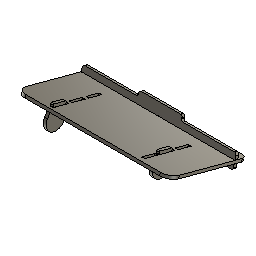
Stand3 (Autodesk Fusion 360 design; units mm, degrees)
Autodesk Fusion 360 part; units mm, degrees
note: some values were not read from the file. Set by a fixed rule: which sketch regions a step uses.
sketch "スケッチ1" plane through (0, 0, 0) normal (0, 0, 1) x (1, 0, 0) in component "base1"
  line L0 (0, 0) -> (160, 0)
  line L1 (160, 0) -> (160, 70)
  line L2 (160, 70) -> (0, 70) construction
  line L3 (0, 70) -> (0, 0)
  line L4 (0, 70) -> (160, 70) construction
  line L5 (160, 70) -> (160, 83)
  line L6 (160, 83) -> (0, 83)
  line L7 (0, 83) -> (0, 70)
  line L8 (80, 70) -> (0, 70)
  line L9 (0, 70) -> (0, 73)
  line L10 (0, 73) -> (80, 73)
  line L11 (80, 73) -> (80, 70)
  line L12 (32, 24) -> (35, 24)
  line L13 (35, 24) -> (35, 38)
  line L14 (35, 38) -> (32, 38)
  line L15 (32, 38) -> (32, 24)
  line L16 (32, 6) -> (35, 6)
  line L17 (35, 6) -> (35, 20)
  line L18 (35, 20) -> (32, 20)
  line L19 (32, 20) -> (32, 6)
  line L20 (125, 6) -> (128, 6)
  line L21 (128, 6) -> (128, 20)
  line L22 (128, 20) -> (125, 20)
  line L23 (125, 20) -> (125, 6)
  line L24 (125, 24) -> (128, 24)
  line L25 (128, 24) -> (128, 38)
  line L26 (128, 38) -> (125, 38)
  line L27 (125, 38) -> (125, 24)
  line L28 (0, 0) -> (32, 6) construction
  line L29 (128, 6) -> (160, 0) construction
  line L30 (32, 56) -> (35, 56)
  line L31 (35, 56) -> (35, 42)
  line L32 (35, 42) -> (32, 42)
  line L33 (32, 42) -> (32, 56)
  line L34 (125, 56) -> (128, 56)
  line L35 (128, 56) -> (128, 42)
  line L36 (128, 42) -> (125, 42)
  line L37 (125, 42) -> (125, 56)
  dimension "d1" = 160
  dimension "d2" = 70
  dimension "d9" = 3
  dimension "d25" = 10
  dimension "d39" = 14
  dimension "d40" = 32
  dimension "d41" = 50
  dimension "d42" = 90
  dimension "d43" = 3
  dimension "d74" = 14
  constraint horizontal L0
  constraint vertical L1
  constraint horizontal L2
  constraint vertical L3
  constraint coincident L0.start L3.end
  constraint horizontal L4
  constraint vertical L5
  constraint horizontal L6
  constraint vertical L7
  constraint coincident L1.end L2.start
  constraint horizontal L8
  constraint vertical L9
  constraint horizontal L10
  constraint vertical L11
  constraint coincident L7 L9.end
  constraint midpoint L2 L8.start
  constraint horizontal L12
  constraint vertical L13
  constraint horizontal L14
  constraint vertical L15
  constraint horizontal L16
  constraint vertical L17
  constraint horizontal L18
  constraint vertical L19
  constraint horizontal L20
  constraint vertical L21
  constraint horizontal L22
  constraint vertical L23
  constraint horizontal L24
  constraint vertical L25
  constraint horizontal L26
  constraint vertical L27
  constraint collinear L16 L20
  constraint collinear L18 L22
  constraint collinear L12 L24
  constraint collinear L14 L26
  constraint equal L12 L16
  constraint equal L16 L20
  constraint equal L20 L24
  constraint collinear L15 L19
  constraint collinear L23 L27
  constraint equal L28 L29
  constraint equal L21 L25
  constraint horizontal L30
  constraint vertical L31
  constraint horizontal L32
  constraint vertical L33
  constraint collinear L15 L33
  constraint collinear L13 L31
  constraint equal L15 L33
  constraint horizontal L34
  constraint vertical L35
  constraint horizontal L36
  constraint vertical L37
  constraint collinear L30 L34
  constraint collinear L32 L36
  constraint collinear L25 L35
  constraint collinear L27 L37
  measures "d1" distance of L0.start L0.end
  measures "d2" distance of L0.start L2.end
  measures "d9" distance of L8.start L10.end
  measures "d25" distance of L6 L10
  measures "d39" distance of L16.start L18.end
  measures "d40" distance of L2.end L14
  measures "d41" vertical distance of L2.end L18.end
  measures "d42" distance of L17.end L22.end
  measures "d43" distance of L16.start L16.end
  measures "d74" vertical distance of L2.end L30.start
extrude "押し出し1" add sketch "スケッチ1" along normal blind 3 contours L0 L1 L3 L5 L6 L7 L8 L10 L11 makes body 1 in component "base1"
sketch "スケッチ1 (2)" plane through (0, 0, 0) normal (0, 1, 0) x (1, 0, 0) in component "back1"
  line L0 (0, 0) -> (-160, 0)
  line L1 (-160, 0) -> (-160, -14)
  line L2 (-160, -14) -> (0, -14)
  line L3 (0, -14) -> (0, 0)
  line L4 (-80, -14) -> (-80, 0) construction
  line L5 (0, -8) -> (-80, -8)
  line L6 (-80, -8) -> (-80, -5)
  line L7 (-80, -5) -> (0, -5)
  line L8 (0, -5) -> (0, -8)
  line L9 (-102.5, -14) -> (-57.5, -14)
  line L10 (-57.5, -14) -> (-57.5, -19)
  line L11 (-57.5, -19) -> (-102.5, -19)
  line L12 (-102.5, -19) -> (-102.5, -14)
  line L13 (-102.5, -19) -> (-160, -14) construction
  line L14 (-57.5, -19) -> (0, -14) construction
  dimension "d10" = 160
  dimension "d11" = 3
  dimension "d18" = 5
  dimension "d20" = 6
  dimension "d26" = 45
  dimension "d28" = 11
  constraint horizontal L0
  constraint vertical L1
  constraint horizontal L2
  constraint vertical L3
  constraint coincident L0.start L3.end
  constraint midpoint L2 L4.start
  constraint midpoint L0 L4.end
  constraint horizontal L5
  constraint vertical L6
  constraint horizontal L7
  constraint vertical L8
  constraint coincident L4 L6.end
  constraint coincident L3 L5.start
  constraint horizontal L9
  constraint vertical L10
  constraint horizontal L11
  constraint vertical L12
  constraint coincident L2 L9.start
  constraint equal L13 L14
  measures "d10" distance of L0.start L0.end
  measures "d11" distance of L5.end L6.end
  measures "d18" distance of L0 L7
  measures "d20" distance of L2 L5
  measures "d26" distance of L9.start L9.end
  measures "d28" distance of L5 L11
extrude "押し出し1'" add sketch "スケッチ1 (2)" along normal blind 3 separate body contours L0 L1 L2 L3 L5 L6 L7 L9 | L2 L9 L10 L11 L12 makes body 2 in component "back1"
fillet "フィレット1" radius 2 4 edges at (-160, 1.5, 0) (-160, 1.5, 14) (0, 1.5, 14) (0, 1.5, 0) on bodies 2 in component "back1"
fillet "フィレット1" radius 2 2 edges at (-102.5, 1.5, 14) (-57.5, 1.5, 14) on bodies 2 in component "back1"
fillet "フィレット1" radius 2 2 edges at (-102.5, 1.5, 19) (-57.5, 1.5, 19) on bodies 2 in component "back1"
fillet "フィレット1'" radius 10 2 edges at (0, 0, 1.5) (160, 0, 1.5) on bodies 1 in component "base1"
fillet "フィレット1'" radius 5 2 edges at (0, 83, 1.5) (160, 83, 1.5) on bodies 1 in component "base1"
sketch "スケッチ1 (3)" plane through (0, 0, 0) normal (1, 0, 0) x (0, 1, 0) in component "leg1"
  line L0 (12.7409, -43.8634) -> (93.405, 23.8218) construction
  line L1 (12.7409, -43.8634) -> (12.7409, -59.189) construction
  circle A0 centre (12.7031, -30.6554) radius 10.1422
  line L2 (2.5609, -30.6554) -> (22.8453, -30.6554)
  line L3 (22.8453, -30.6554) -> (22.8453, -19.5375)
  line L4 (2.5609, -24.9727) -> (2.5609, -30.6554)
  line L5 (2.5609, -24.9727) -> (22.8453, -19.5375)
  line L6 (4.4927, -24.4551) -> (2.9398, -18.6595)
  line L7 (2.9398, -18.6595) -> (16.4628, -15.0361)
  line L8 (16.4628, -15.0361) -> (18.0157, -20.8316)
  line L9 (7.3905, -23.6786) -> (6.614, -20.7809)
  line L10 (6.614, -20.7809) -> (3.7163, -21.5573)
  dimension "d44" = 130
  dimension "d46" = 3
  dimension "d47" = 3
  dimension "d48" = 14
  dimension "d49" = 15
  dimension "d59" = 3
  dimension "d61" = 5
  dimension "d62" = 2
  constraint vertical L1
  constraint horizontal L2
  constraint tangent A0 L3
  constraint tangent L0 A0
  constraint perpendicular L6 L7
  constraint perpendicular L7 L8
  constraint coincident L5 L9.start
  constraint perpendicular L5 L9
  constraint coincident L6 L10.end
  constraint perpendicular L5 L8
  constraint perpendicular L9 L10
  constraint parallel L3 L4
  constraint coincident L8.end L5
  constraint coincident L6.start L5
  constraint coincident A0 L2.end
  constraint coincident A0 L2.start
  constraint tangent A0 L4
  measures "d44" angle of L0 L1
  measures "d46" distance of L9.start L9.end
  measures "d47" distance of L6.end L10.end
  measures "d48" distance of L6.end L7.end
  measures "d49" angle of L3 L8
  measures "d59" distance of L9.end L10.end
  measures "d61" distance of L8 L3.end
  measures "d62" distance of L6 L4.start
extrude "押し出し1''" add sketch "スケッチ1 (3)" along normal blind 3 separate body contours A0 L2 | A0 L4 L5 | A0 L2 L5 | A0 L3 L5 | A0 L5 L9 | A0 L5 L6 L7 L8 L9 L10 picked at (7.5453, -22.4968) makes body 3 in component "leg1"
fillet "フィレット1''" radius 1 2 edges at (1.5, 2.9398, -18.6595) (1.5, 16.4628, -15.0361) on bodies 3 in component "leg1"
fillet "フィレット1''" radius 0.5 2 edges at (1.5, 3.7163, -21.5573) (1.5, 2.5609, -24.9727) on bodies 3 in component "leg1"
fillet "フィレット1''" radius 0.5 1 edges at (1.5, 22.8453, -19.5375) on bodies 3 in component "leg1"
component "stand1" placed x (1, 0, 0) y (0, 0.766044, -0.642788) z (0, 0.642788, 0.766044) at (0, 0, 0)
component "base1" placed x (1, 0, 0) y (0, 0.906308, 0.422618) z (0, -0.422618, 0.906308) at (60, 5.8917, -23.5756) in component "stand1"
component "back1" placed x (1, 0, 0) y (0, 0.906308, 0.422618) z (0, -0.422618, 0.906308) at (220, 71.4463, 1.4761) in component "stand1"
component "leg1" placed x (1, 0, 0) y (0, 0.984808, 0.173648) z (0, -0.173648, 0.984808) at (92, -0.0605, 0.9956) in component "stand1"
component "leg1" placed x (1, 0, 0) y (0, 0.984808, 0.173648) z (0, -0.173648, 0.984808) at (185, 16.2531, 8.6028) in component "stand1"
equation "d1 = width1"
equation "d2 = depth1"
equation "width1 = 160 mm"
equation "depth1 = 70 mm"
equation "thickness1 = 3 mm"
equation "d7 = thickness1"
equation "d9 = thickness1"
equation "d10 = width1"
equation "d11 = thickness1"
equation "d12 = thickness1"
equation "d43 = thickness1"
equation "d46 = thickness1"
equation "d48 = d39"
equation "d51 = thickness1"
equation "d61 = d59 + 2 mm"
